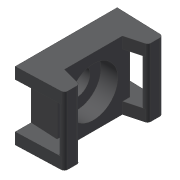
# Autodesk Inventor part: 520022598
Saved by Autodesk Inventor 2021.3 (Build 253353000, 353)
## iProperties
Category: PARTsolutions
Company: BOSSARD
Manager: SROAMA
Created: 2013-12-10
Part Number: 520022598
Catalog Web Link: www.cadenas.de
Description: Kabelbindersockel M3 Pa 6.6 schw BN20343
Vendor: BOSSARD
Document SubType Name: Modeling
Designer: SROSL
Manufacturer: BOSSARD
Density: 1.6 g/cm^3
Mass: 0.699988 g
Surface Area: 6.87016 cm^2
Volume: 0.437493 cm^3
Project: Peiros
User Status: Schnelländerung
Material: PA 6.6-MO*Nylatron GS
Engineer: SROSL
Appearance: RGB(35.70000015199275,35.70000015199275,35.70000015199275)
PSOL_IDENT_0: {$CADENAS_DATA\23d-libs\bossard\13\13_20\13_20_90\bn_20342_20343\bn_20343.prj},212 {VTYP=3D},{NB=BN
PSOL_IDENT_1: 20343 3389411 cable tie mount 5},{LINA=BN 20343 3389411 cable tie mount 5},{NN=BN 20343},{DATE=04.12
PSOL_IDENT_2: .2012 11:45:29},{GEOMDATE=06.07.2012 07:21:53},{VERSION=},{LINEID=10},{LINESUBID=-1},{WBVAR=}  {NB=B
PSOL_IDENT_3: N 20343 3389411 cable tie mount 5},{LINA=BN 20343 3389411 cable tie mount 5},{KT=DUMMY},{NENN=5},{CN
PSOL_IDENT_4: SORDERNO=3389411},{BNARTNR=3389411},{BNNORM1=},{BNMAT=Polyamid PA 6.6},{CNSMAT=Polyamid PA 6.6},{BNS
PSOL_IDENT_5: URFACE=schwarz},{D1=5},{D11=3.000},{A=15},{B=10},{C=7},{R1=0.500},{R2=0.500},{R3=0.500},{R4=0.500}
CNS_NN: BN 20343
CNS_NT: Cable tie mounts, black
CNS_NB: BN 20343 3389411 cable tie mount 5
CNS_NBSYN: BN 20343 $BNARTNR. cable tie mount $NENN.
CNS_LINA: BN 20343 3389411 cable tie mount 5
CNS_ROWDESC: 5
CNS_NENN: 5
CNS_CNSORDERNO: 3389411
CNS_BNARTNR: 3389411
CNS_BNMAT: Polyamide PA 6.6
CNS_CNSMAT: Polyamide PA 6.6
CNS_BNSURFACE: black
CNS_D1: 5
CNS_D11: 3.000
CNS_A: 15
CNS_B: 10
CNS_C: 7
CNS_R1: 0.500
CNS_R2: 0.500
CNS_R3: 0.500
CNS_R4: 0.500
SUPPLIER: BOSSARD
ARTICLENO: BN 20343 3389411 cable tie mount 5
BOMINFO: BN 20343 3389411 cable tie mount 5
CREATOR: CADENAS GmbH
Dateiname: 520_022_598
Zeichnungsnummer: 520022598
Zeichnungsname: 520 022 598
Titel: Kabelbindersockel M3 Pa 6.6 Schwarz
Status: Freigegeben
Erstellt_am: 10.12.2013
Erstellt_durch: SL
Freigegeben_am: 20.01.2014
Freigegeben_durch: HEJ
Material_Werkstoffnummer: PA 6.6-MO
Material_Bezeichnung: Nylatron GS
Gewicht: 0.001 kg
DOCID: 109804
PDB_IDENT: 520022598
PDB_Name: 520022598
PDB_Ident_Ver: =<PDB_Ident> <PDB_Version>
STID: 26026
PDB_Mat: Nylatron GS
ROT_Weight: 0.001 kg
ROT_Weight_Num: 0.0006999880710171054
Title: Kabelbindersockel M3 Pa 6.6 schw BN20343
Author: SROSL
Comments: Cable tie mounts, black
Autodesk Inventor part; units mm, degrees
ref_plane "YZ Plane" through (0, 0, 0) normal (1, 0, 0) x (0, 1, 0)
ref_plane "XZ Plane" through (0, 0, 0) normal (0, 1, 0) x (-1, 0, 0)
ref_plane "XY Plane" through (0, 0, 0) normal (0, 0, 1) x (1, 0, 0)
sketch "Sketch_1" plane through (0, 0, 0) normal (0, 0, 1) x (1, 0, 0)
  line L0 (0, 7.5) -> (0, -7.5)
  line L1 (0, -7.5) -> (6.5174, -7.2724)
  arc A0 (6.5174, -7.2724) -> (7, -6.7727) centre (6.5, -6.7727) ccw
  line L2 (7, -6.7727) -> (7, -5.4555)
  arc A1 (7, -5.4555) -> (6.6294, -4.9725) centre (6.5, -5.4555) ccw
  line L3 (6.6294, -4.9725) -> (4, -4.2679)
  line L4 (4, -4.2679) -> (4, 4.2679)
  line L5 (4, 4.2679) -> (6.6294, 4.9725)
  arc A2 (6.6294, 4.9725) -> (7, 5.4555) centre (6.5, 5.4555) ccw
  line L6 (7, 5.4555) -> (7, 6.7727)
  arc A3 (7, 6.7727) -> (6.5174, 7.2724) centre (6.5, 6.7727) ccw
  line L7 (6.5174, 7.2724) -> (0, 7.5)
  point P0 (0, 0)
  point P1 (0, 0)
  dimension "d11" = 4
  constraints: 16 end point, 8 point on circle, 4 centre point, 2 vertical, 1 coincident, 1 midpoint, 20 other
  measures "d11" distance between parallel lines of L4 L0
extrude "Extrusion1" add sketch "Sketch_1" along normal mid plane 10
sketch "Sketch_3" plane through (0, 0, 0) normal (0, 0, 1) x (1, 0, 0)
  line L0 (0, 8.3333) -> (0, 5.141)
  line L1 (0, 5.141) -> (4, 5.3458)
  line L2 (4, 5.3458) -> (4, 0)
  line L3 (4, 0) -> (8, 0)
  line L4 (8, 0) -> (8, 8.3333)
  line L5 (8, 8.3333) -> (0, 8.3333)
  arc A0 (6, 5.4555) -> (6.6294, 4.9725) centre (6.5, 5.4555) ccw
  arc A1 (6.6294, 4.9725) -> (7, 5.4555) centre (6.5, 5.4555) ccw
  line L6 (7, 5.4555) -> (7, 6.7727)
  arc A2 (7, 6.7727) -> (6.5174, 7.2724) centre (6.5, 6.7727) ccw
  arc A3 (6.5174, 7.2724) -> (6, 6.7727) centre (6.5, 6.7727) ccw
  line L7 (6, 6.7727) -> (6, 5.4555)
  line L8 (4, -4.2679) -> (4, 4.2679) projected
  line L9 (0, 7.5) -> (0, -7.5) projected
  constraints: 16 end point, 8 point on circle, 4 centre point, 4 vertical, 2 horizontal, 1 midpoint, 1 point on line, 16 other
extrude "Extrusion2" cut sketch "Sketch_3" along normal mid plane 6.6667
sketch "Sketch_4" plane through (0, 0, 0) normal (0, 0, 1) x (1, 0, 0)
  line L0 (0, -8.3333) -> (8, -8.3333)
  line L1 (8, -8.3333) -> (8, 0)
  line L2 (8, 0) -> (4, 0)
  line L3 (4, 0) -> (4, -5.3506)
  line L4 (4, -5.3506) -> (0, -5.141)
  line L5 (0, -5.141) -> (0, -8.3333)
  line L6 (6, -5.4555) -> (6, -6.7727)
  arc A0 (6, -6.7727) -> (6.5174, -7.2724) centre (6.5, -6.7727) ccw
  arc A1 (6.5174, -7.2724) -> (7, -6.7727) centre (6.5, -6.7727) ccw
  line L7 (7, -6.7727) -> (7, -5.4555)
  arc A2 (7, -5.4555) -> (6.6294, -4.9725) centre (6.5, -5.4555) ccw
  arc A3 (6.6294, -4.9725) -> (6, -5.4555) centre (6.5, -5.4555) ccw
  line L8 (4, -4.2679) -> (4, 4.2679) projected
  line L9 (0, 7.5) -> (0, -7.5) projected
  constraints: 16 end point, 8 point on circle, 4 centre point, 4 vertical, 2 horizontal, 1 midpoint, 16 other
extrude "Extrusion3" cut sketch "Sketch_4" along normal mid plane 6.6667
sketch "Sketch_5" plane through (0, 0, 0) normal (0, 0, 1) x (1, 0, 0)
  line L0 (4, 0) -> (0, 0)
  line L1 (0, 0) -> (0, 2)
  line L2 (0, 2) -> (1.5, 2)
  line L3 (1.5, 2) -> (1.5, 3.6)
  line L4 (1.5, 3.6) -> (4, 3.6)
  line L5 (4, 3.6) -> (4, 0)
  line L6 (4, 0) -> (0, 0)
  line L7 (7, 5.4555) -> (7, 6.7727) projected
  line L8 (4, -4.2679) -> (4, 4.2679) projected
  line L9 (0, 7.5) -> (0, -7.5) projected
  dimension "d7" = 2
  dimension "d8" = 3.6
  dimension "d9" = 5.5
  constraints: 14 end point, 2 midpoint, 2 vertical, 1 horizontal
  measures "d7" distance between parallel lines of L2 L0
  measures "d8" distance between parallel lines of L4 L0
  measures "d9" distance between parallel lines of L7 L3
revolve "Revolution1" cut sketch "Sketch_5" angle 360 about axis through (4, 0, 0) along (1, 0, 0)
body "Solid1"
